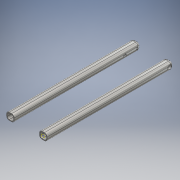
# Autodesk Inventor part: astabella_lunga
Saved by Autodesk Inventor 2016 (Build 200138000, 138)
## iProperties
Created: 2017-09-06
Part Number: astabella_lunga
Material: Aluminum 6061
Document SubType Name: Modeling
Designer: Davide
Density: 2.7 g/cm^3
Appearance: Aluminum - Polished
Mass: 351.143 g
Surface Area: 346.176 cm^2
Volume: 130.053 cm^3
Author: Davide
Autodesk Inventor part; units mm, degrees
ref_plane "YZ Plane" through (0, 0, 0) normal (1, 0, 0) x (0, 1, 0)
ref_plane "XZ Plane" through (0, 0, 0) normal (0, 1, 0) x (-1, 0, 0)
ref_plane "XY Plane" through (0, 0, 0) normal (0, 0, 1) x (1, 0, 0)
sketch "Sketch1" plane through (0, 0, 0) normal (0, 0, 1) x (1, 0, 0)
  line L0 (-25, 0) -> (25, 0)
  line L1 (25, 0) -> (25, 28)
  line L2 (25, 28) -> (-25, 28)
  line L3 (-25, 28) -> (-25, 0)
  line L4 (25, 14) -> (40, 14)
  line L5 (40, 14) -> (40, 314)
  line L6 (40, 314) -> (25, 314)
  line L7 (25, 314) -> (25, 14)
  line L8 (-25, 14) -> (-40, 14)
  line L9 (-40, 14) -> (-40, 314)
  line L10 (-40, 314) -> (-25, 314)
  line L11 (-25, 314) -> (-25, 14)
  point P0 (0, 0)
  point P1 (0, 0)
  dimension "d0" = 50
  dimension "d1" = 15
  dimension "d2" = 15
  dimension "d3" = 28
  dimension "d4" = 300
  dimension "d5" = 300
  constraints: 24 end point, 6 parallel, 3 horizontal, 3 midpoint, 3 perpendicular, 1 coincident, 1 collinear
  measures "d0" distance of L1.end L2.end
  measures "d1" distance of L9.end L10.end
  measures "d2" distance of L5.end L6.end
  measures "d3" distance of L0.end L1.end
  measures "d4" distance of L4.end L5.end
  measures "d5" distance of L8.end L9.end
extrude "Extrusion1" add sketch "Sketch1" along normal blind 14
fillet "Fillet1" radius 5 36 edges at (25, 28, 7) (25, 171, 14) (25, 314, 7) (25, 171, 0) (32.5, 314, 0) (32.5, 314, 14) (40, 314, 7) (40, 164, 0) (40, 164, 14) (40, 14, 7) (32.5, 14, 0) (32.5, 14, 14) (25, 14, 7) (-25, 28, 7) (-25, 171, 0) (-25, 314, 7) (-25, 171, 14) (-32.5, 14, 0) (-25, 14, 7) (-32.5, 14, 14) (-40, 14, 7) (-40, 164, 0) (-40, 164, 14) (-40, 314, 7) (-32.5, 314, 0) (-32.5, 314, 14) (-25, 7, 0) (-25, 0, 7) (-25, 7, 14) (0, 28, 0) (0, 28, 14) (25, 7, 14) (25, 0, 7) (25, 7, 0) (0, 0, 0) (0, 0, 14)
sketch "Sketch2" plane through (25, 5, 5) normal (1, 0, 0) x (0, 0, -1)
  line L0 (-9, 4) -> (-9, 0) projected
  line L1 (-4, -5) -> (0, -5) projected
  line L2 (5, 0) -> (5, 4) projected
  circle A0 centre (-2, 2) radius 7 construction
  circle A1 centre (-2, 2) radius 2
  point P0 (5, -5)
  dimension "d9" = 4
  constraints: 3 tangent, 2 centre point, 1 coincident
  measures "d9" diameter of A1
extrude "Extrusion2" cut sketch "Sketch2" against normal through all
sketch "Sketch3" plane through (40, 19, 5) normal (1, 0, 0) x (0, 0, -1)
  line L0 (0, 0) -> (0, 290) projected
  line L1 (0, 290) -> (-4, 290) projected
  line L2 (-4, 0) -> (-4, 290) projected
  line L3 (0, 0) -> (-4, 0) projected
  line L4 (-9, 290) -> (-9, 0) projected
  line L5 (0, 295) -> (-4, 295) projected
  line L6 (5, 0) -> (5, 290) projected
  circle A0 centre (-2, 288) radius 7 construction
  circle A1 centre (-2, 288) radius 2
  circle A2 centre (-2, 288) radius 4
  point P0 (5, -19)
  dimension "d12" = 4
  dimension "d44" = 8
  constraints: 3 centre point, 3 tangent, 2 coincident
  measures "d12" diameter of A1
  measures "d44" diameter of A2
extrude "Extrusion3" cut sketch "Sketch3" against normal through all contours A1
ref_plane "Work Plane1" through (30, 294, 5) normal (0, 1, 0) x (1, 0, 0)
sketch "Sketch4" plane through (30, 294, 5) normal (0, 1, 0) x (1, 0, 0)
  arc A0 (5, -9) -> (10, -4) centre (5, -4) ccw projected
  line L0 (10, -4) -> (10, -2) projected
  line L1 (10, -2) -> (10, 0) projected
  arc A1 (10, 0) -> (5, 5) centre (5, 0) ccw projected
  line L2 (5, 5) -> (0, 5) projected
  arc A2 (0, 5) -> (-5, 0) centre (0, 0) ccw projected
  line L3 (-5, 0) -> (-5, -2) projected
  line L4 (-5, -2) -> (-5, -4) projected
  arc A3 (-5, -4) -> (0, -9) centre (0, -4) ccw projected
  line L5 (0, -9) -> (5, -9) projected
  arc A4 (5, -7.5) -> (8.5, -4) centre (5, -4) ccw
  line L6 (8.5, -4) -> (8.5, -2)
  line L7 (8.5, -2) -> (8.5, 0)
  arc A5 (8.5, 0) -> (5, 3.5) centre (5, 0) ccw
  line L8 (5, 3.5) -> (0, 3.5)
  arc A6 (0, 3.5) -> (-3.5, 0) centre (0, 0) ccw
  line L9 (-3.5, 0) -> (-3.5, -2)
  line L10 (-3.5, -2) -> (-3.5, -4)
  arc A7 (-3.5, -4) -> (0, -7.5) centre (0, -4) ccw
  line L11 (0, -7.5) -> (5, -7.5)
  arc A8 (-60, -9) -> (-55, -4) centre (-60, -4) ccw projected
  line L12 (-65, -9) -> (-60, -9) projected
  arc A9 (-70, -4) -> (-65, -9) centre (-65, -4) ccw projected
  line L13 (-70, 0) -> (-70, -2) projected
  line L14 (-70, -2) -> (-70, -4) projected
  arc A10 (-65, 5) -> (-70, 0) centre (-65, 0) ccw projected
  line L15 (-60, 5) -> (-65, 5) projected
  arc A11 (-55, 0) -> (-60, 5) centre (-60, 0) ccw projected
  line L16 (-55, -2) -> (-55, 0) projected
  line L17 (-55, -4) -> (-55, -2) projected
  arc A12 (-60, -7.5) -> (-56.5, -4) centre (-60, -4) ccw
  line L18 (-60, -7.5) -> (-65, -7.5)
  arc A13 (-68.5, -4) -> (-65, -7.5) centre (-65, -4) ccw
  line L19 (-68.5, -4) -> (-68.5, -2)
  line L20 (-68.5, -2) -> (-68.5, 0)
  arc A14 (-65, 3.5) -> (-68.5, 0) centre (-65, 0) ccw
  line L21 (-65, 3.5) -> (-60, 3.5)
  arc A15 (-56.5, 0) -> (-60, 3.5) centre (-60, 0) ccw
  line L22 (-56.5, 0) -> (-56.5, -2)
  line L23 (-56.5, -2) -> (-56.5, -4)
  point P0 (-30, 5)
  dimension "d16" = 1.5
  dimension "d17" = 1.5
  constraints: 24 end point, 16 point on circle, 8 centre point, 18 other
  measures "d16" distance between parallel lines of L5 L11
  measures "d17" distance between parallel lines of L12 L18
extrude "Extrusion4" cut sketch "Sketch4" against normal blind 250 contours L11 A7 L10 L9 A6 L8 A5 L7 L6 A4 | L18 A13 L19 L20 A14 L21 A15 L22 L23 A12
sketch "Sketch5" plane through (-25, 33, 9) normal (1, 0, 0) x (0, 0, -1)
  line L0 (4, 0) -> (0, 0) projected
  line L1 (2, 0) -> (2, 11.8372) construction
  circle A0 centre (2, 20) radius 2.5
  circle A1 centre (2, 250) radius 2.5
  point P0 (9, -33)
  dimension "d20" = 5
  dimension "d21" = 20
  dimension "d24" = 230
  constraints: 2 centre point, 2 end point, 2 vertical, 1 midpoint, 1 point on line, 2 other
  measures "d20" diameter of A0
  measures "d21" distance of A0.centre L1.start
  measures "d24" distance of A0.centre A1.centre
extrude "Extrusion5" cut sketch "Sketch5" against normal up to next
ref_plane "Work Plane2" through (30, 194, 5) normal (0, 1, 0) x (1, 0, 0)
ref_plane "Work Plane3" through (30, 64, 5) normal (0, 1, 0) x (1, 0, 0)
split "Split2" plane through (30, 64, 5) removes the side toward (0, -1, 0)
sketch "Sketch7" plane through (-35, 64, 14) normal (0, -1, 0) x (1, 0, 0)
  arc A0 (65, -1.5) -> (61.5, -5) centre (65, -5) ccw projected
  line L0 (61.5, -5) -> (61.5, -9) projected
  arc A1 (61.5, -9) -> (65, -12.5) centre (65, -9) ccw projected
  line L1 (65, -12.5) -> (70, -12.5) projected
  arc A2 (70, -12.5) -> (73.5, -9) centre (70, -9) ccw projected
  line L2 (73.5, -9) -> (73.5, -5) projected
  arc A3 (73.5, -5) -> (70, -1.5) centre (70, -5) ccw projected
  line L3 (70, -1.5) -> (65, -1.5) projected
  line L4 (70, -14) -> (65, -14) projected
  arc A4 (60, -9) -> (65, -14) centre (65, -9) ccw projected
  line L5 (60, -9) -> (60, -5) projected
  arc A5 (65, 0) -> (60, -5) centre (65, -5) ccw projected
  line L6 (65, 0) -> (70, 0) projected
  arc A6 (75, -5) -> (70, 0) centre (70, -5) ccw projected
  line L7 (75, -5) -> (75, -9) projected
  arc A7 (70, -14) -> (75, -9) centre (70, -9) ccw projected
  arc A8 (0, -1.5) -> (-3.5, -5) centre (0, -5) ccw projected
  line L8 (-3.5, -5) -> (-3.5, -9) projected
  arc A9 (-3.5, -9) -> (0, -12.5) centre (0, -9) ccw projected
  line L9 (0, -12.5) -> (5, -12.5) projected
  arc A10 (5, -12.5) -> (8.5, -9) centre (5, -9) ccw projected
  line L10 (8.5, -9) -> (8.5, -5) projected
  arc A11 (8.5, -5) -> (5, -1.5) centre (5, -5) ccw projected
  line L11 (5, -1.5) -> (0, -1.5) projected
  line L12 (0, 0) -> (5, 0) projected
  arc A12 (10, -5) -> (5, 0) centre (5, -5) ccw projected
  line L13 (10, -5) -> (10, -9) projected
  arc A13 (5, -14) -> (10, -9) centre (5, -9) ccw projected
  line L14 (5, -14) -> (0, -14) projected
  arc A14 (-5, -9) -> (0, -14) centre (0, -9) ccw projected
  line L15 (-5, -9) -> (-5, -5) projected
  arc A15 (0, 0) -> (-5, -5) centre (0, -5) ccw projected
  arc A16 (0, -1.5) -> (-3.5, -5) centre (0, -5) ccw projected
  line L16 (5, -1.5) -> (0, -1.5) projected
  arc A17 (8.5, -5) -> (5, -1.5) centre (5, -5) ccw projected
  line L17 (8.5, -9) -> (8.5, -5) projected
  arc A18 (5, -12.5) -> (8.5, -9) centre (5, -9) ccw projected
  line L18 (0, -12.5) -> (5, -12.5) projected
  arc A19 (-3.5, -9) -> (0, -12.5) centre (0, -9) ccw projected
  line L19 (-3.5, -5) -> (-3.5, -9) projected
  line L20 (-3.7, -5) -> (-3.7, -9)
  arc A20 (-3.7, -9) -> (0, -12.7) centre (0, -9) ccw
  line L21 (0, -12.7) -> (5, -12.7)
  arc A21 (5, -12.7) -> (8.7, -9) centre (5, -9) ccw
  line L22 (8.7, -9) -> (8.7, -5)
  arc A22 (8.7, -5) -> (5, -1.3) centre (5, -5) ccw
  line L23 (5, -1.3) -> (0, -1.3)
  arc A23 (0, -1.3) -> (-3.7, -5) centre (0, -5) ccw
  line L24 (61.3, -5) -> (61.3, -9)
  arc A24 (61.3, -9) -> (65, -12.7) centre (65, -9) ccw
  line L25 (65, -12.7) -> (70, -12.7)
  arc A25 (70, -12.7) -> (73.7, -9) centre (70, -9) ccw
  line L26 (73.7, -9) -> (73.7, -5)
  arc A26 (73.7, -5) -> (70, -1.3) centre (70, -5) ccw
  line L27 (70, -1.3) -> (65, -1.3)
  arc A27 (65, -1.3) -> (61.3, -5) centre (65, -5) ccw
  point P0 (35, -14)
  dimension "d40" = 0.2
  dimension "d41" = 0.2
  constraints: 16 end point, 16 point on circle, 8 centre point, 14 other
  measures "d40" distance between parallel lines of L8 L20
  measures "d41" distance between parallel lines of L24 L0
extrude "Extrusion8" cut sketch "Sketch7" against normal blind 15 contours A23 L23 A22 L22 A21 L21 A20 L20 | A27 L27 A26 L26 A25 L25 A24 L24
extrude "Extrusion9" cut sketch "Sketch3" against normal blind 4 contours A1 L1 L0 | L0 L1 L2 A2 | L0 A2 L2 A1 | A1 L2 L1
mirror "Mirror1" about plane through (0, 0, 0) normal (1, 0, 0) of "Extrusion9"
equation "\"d2\" = d1"
equation "\"d5\" = d4"
equation "\"d10\" = d9"
equation "\"d17\" = d16"
equation "\"d41\" = d40"
body "Solid1"
